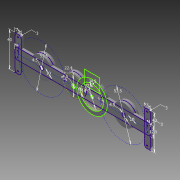
# Autodesk Inventor part: OuterBar
Saved by Autodesk Inventor 2014 SP1 (Build 180222100, 222)
## iProperties
Created: 2014-06-07
Part Number: OuterBar
Material: Generic
Document SubType Name: Modeling
Designer: Erin
Density: 1 g/cm^3
Appearance: Default
Author: Erin
Autodesk Inventor part; units mm, degrees
note: some values were not read from the file. Chosen so that the rebuilt part matches the saved one: sketch regions of "Extrusion1".
ref_plane "YZ Plane" through (0, 0, 0) normal (1, 0, 0) x (0, 1, 0)
ref_plane "XZ Plane" through (0, 0, 0) normal (0, 1, 0) x (-1, 0, 0)
ref_plane "XY Plane" through (0, 0, 0) normal (0, 0, 1) x (1, 0, 0)
sketch "Sketch1" plane through (0, 0, 0) normal (0, 1, 0) x (-1, 0, 0)
  line L0 (-75.4, 6.25) -> (75.4, 6.25)
  line L1 (78.4, 3.25) -> (78.4, -3.25)
  line L2 (75.4, -6.25) -> (-75.4, -6.25)
  line L3 (-78.4, -3.25) -> (-78.4, 3.25)
  circle A0 centre (-47.65, 0) radius 2.25
  circle A1 centre (47.65, 0) radius 2.25
  circle A2 centre (-47.65, 0) radius 26.75 construction
  circle A3 centre (-10.7, 0) radius 1.7
  circle A4 centre (-10.7, 0) radius 11.2 construction
  line L4 (-21.9, 0) -> (-21.9, 5.3604)
  line L5 (-20.9, 0) -> (-20.9, 5.3604)
  circle A5 centre (10.7, 0) radius 2.25
  circle A6 centre (10.7, 0) radius 11.2 construction
  line L6 (-0.5, 0) -> (-0.5, 4.194)
  line L7 (0.5, 0) -> (0.5, 4.194)
  circle A7 centre (47.65, 0) radius 26.75 construction
  line L8 (20.9, 0) -> (20.9, 4.3426)
  line L9 (21.9, 0) -> (21.9, 4.3426)
  arc A8 (-75.4, 6.25) -> (-78.4, 3.25) centre (-75.4, 3.25) ccw
  arc A9 (-78.4, -3.25) -> (-75.4, -6.25) centre (-75.4, -3.25) ccw
  arc A10 (78.4, 3.25) -> (75.4, 6.25) centre (75.4, 3.25) ccw
  arc A11 (75.4, -6.25) -> (78.4, -3.25) centre (75.4, -3.25) ccw
  line L10 (-81.9483, 0) -> (78.4, 0) construction
  circle A12 centre (-10.7, 0) radius 13.2
  circle A13 centre (-10.7, 0) radius 17.7
  line L11 (74.4, 0) -> (74.4, 11.2)
  line L12 (-74.4, 0) -> (-74.4, 10)
  line L13 (-75.4, 20) -> (-74.4, 20)
  line L14 (-71.4, 17) -> (-71.4, -17)
  line L15 (-74.4, -20) -> (-75.4, -20)
  line L16 (-78.4, -17) -> (-78.4, 17)
  line L17 (75.4, 20) -> (74.4, 20)
  line L18 (71.4, 17) -> (71.4, -17)
  line L19 (74.4, -20) -> (75.4, -20)
  line L20 (78.4, -17) -> (78.4, 17)
  arc A14 (74.4, 20) -> (71.4, 17) centre (74.4, 17) ccw
  arc A15 (78.4, 17) -> (75.4, 20) centre (75.4, 17) ccw
  arc A16 (75.4, -20) -> (78.4, -17) centre (75.4, -17) ccw
  arc A17 (71.4, -17) -> (74.4, -20) centre (74.4, -17) ccw
  arc A18 (-75.4, 20) -> (-78.4, 17) centre (-75.4, 17) ccw
  arc A19 (-71.4, 17) -> (-74.4, 20) centre (-74.4, 17) ccw
  arc A20 (-74.4, -20) -> (-71.4, -17) centre (-74.4, -17) ccw
  arc A21 (-78.4, -17) -> (-75.4, -20) centre (-75.4, -17) ccw
  line L21 (-19.3726, 23.4692) -> (-1.7741, 23.4692)
  line L22 (-1.7741, 23.4692) -> (-1.7741, 7.4894)
  line L23 (-1.7741, 7.4894) -> (-19.3726, 7.4894)
  line L24 (-19.3726, 7.4894) -> (-19.3726, 23.4692)
  point P0 (0, 0)
  point P1 (-78.4, 6.25)
  point P2 (-78.4, -6.25)
  point P3 (0, 6.25)
  point P4 (-78.4, 20)
  point P5 (-71.4, 20)
  point P6 (-78.4, -20)
  point P7 (-78.4, 0)
  point P8 (-78.4, 0)
  point P9 (78.4, 20)
  point P10 (71.4, 20)
  point P11 (78.4, -20)
  point P12 (78.4, 0)
  dimension "d0" = 12.5
  dimension "d1" = 4.5
  dimension "d3" = 4.5
  dimension "d5" = 53.5
  dimension "d6" = 3.4
  dimension "d7" = 22.4
  dimension "d8" = 1
  dimension "d9" = 4.5
  dimension "d10" = 22.4
  dimension "d11" = 1
  dimension "d12" = 53.5
  dimension "d13" = 1
  dimension "d14" = 3
  dimension "d23" = 4.5
  dimension "d26" = 4
  dimension "d27" = 4
  dimension "d28" = 7
  dimension "d29" = 40
  dimension "d30" = 7
  dimension "d31" = 40
  dimension "d32" = 3
  dimension "d33" = 3
  dimension "d39" = 2
  constraints: 50 end point, 32 point on circle, 32 tangent, 22 centre point, 19 point on line, 15 parallel, 9 equal radius, 8 coincident, 6 perpendicular, 5 horizontal, 5 midpoint, 2 collinear, 1 horizontal alignment, 1 vertical alignment
  measures "d0" distance of point (-78.4, -6.25) point (-78.4, 6.25)
  measures "d1" diameter of A0
  measures "d3" diameter of A1
  measures "d5" diameter of A2
  measures "d6" diameter of A3
  measures "d7" diameter of A4
  measures "d8" distance between parallel lines of L5 L4
  measures "d9" diameter of A5
  measures "d10" diameter of A6
  measures "d11" distance between parallel lines of L7 L6
  measures "d12" diameter of A7
  measures "d13" distance between parallel lines of L9 L8
  measures "d14" radius of A8
  measures "d23" radial gap between concentric circles of A12 A13
  measures "d26" distance between parallel lines of L11 L1
  measures "d27" distance between parallel lines of L12 L3
  measures "d28" distance of point (-78.4, 20) point (-71.4, 20)
  measures "d29" distance of point (-78.4, -20) point (-78.4, 20)
  measures "d30" distance of point (78.4, 20) point (71.4, 20)
  measures "d31" distance of point (78.4, -20) point (78.4, 20)
  measures "d32" radius of A14
  measures "d33" radius of A18
  measures "d39" radial gap between concentric circles of A4 A12
extrude "Extrusion1" add sketch "Sketch1" along normal blind 3 contours A8 L16 A18 L13 A19 L14 L0 | L0 L14 L2 A9 L3 A8 | L0 A13 L2 L14 | A9 L2 L14 A20 L15 A21 L16 | A13 L24 A12 L0 | L0 A12 L2 A13 | A13 L22 A12 L24 | L2 A12 A13 | A12 L22 A13 L0 | L0 A13 L2 A12 | A13 L0 L18 L2 | L18 L0 A10 L1 A11 L2 | L2 A11 L20 A16 L19 A17 L18 | L18 A14 L17 A15 L20 A10 L0
extrude "Extrusion2" cut sketch "Sketch1" along normal blind 10 contours A12 L24 L23 L22 L0 | L0 A12 L2 | A12 L22 L23 L24 | L2 A12
sketch "Sketch2" plane through (0, 3, 0) normal (0, 1, 0) x (1, 0, 0)
  circle A0 centre (47.65, 0) radius 2.25 projected
  circle A1 centre (-10.7, 0) radius 2.25 projected
  circle A2 centre (-47.65, 0) radius 2.25 projected
  circle A3 centre (-47.65, 0) radius 12.25
  circle A4 centre (-10.7, 0) radius 12.25
  circle A5 centre (47.65, 0) radius 12.25
  point P0 (0, 0)
  dimension "d34" = 10
  dimension "d35" = 10
  dimension "d36" = 10
  constraints: 3 centre point, 3 coincident
  measures "d34" radial gap between concentric circles of A2 A3
  measures "d35" radial gap between concentric circles of A1 A4
  measures "d36" radial gap between concentric circles of A0 A5
extrude "Extrusion3" add sketch "Sketch2" along normal blind 3
extrude "Extrusion4" cut sketch "Sketch1" along normal blind 3 contours L24 L21 L22 A13 | A13 L22 A12 L24 | A12 L22 L23 L24
extrude "Extrusion5" add sketch "Sketch2" against normal blind 3
extrude "Extrusion6" cut sketch "Sketch1" along normal mid plane 20 contours A12 L24 L23 L22 L0 | L0 A12 L2 | A12 L22 L23 L24 | L2 A12
equation "\"sp\" = 0.4"
body "Solid1"
